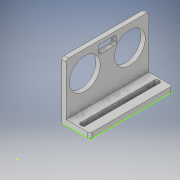
# Autodesk Inventor part: UltrasonicSensorMountSingle
Saved by Autodesk Inventor 2019 (Build 230136000, 136)
## iProperties
Created: 2020-06-23
Part Number: UltrasonicSensorMountSingle
Material: Generic
Document SubType Name: Modeling
Designer: garretthagen21
Density: 1 g/cm^3
Appearance: Default
Author: garretthagen21
Autodesk Inventor part; units mm, degrees
ref_plane "YZ Plane" through (0, 0, 0) normal (1, 0, 0) x (0, 1, 0)
ref_plane "XZ Plane" through (0, 0, 0) normal (0, 1, 0) x (-1, 0, 0)
ref_plane "XY Plane" through (0, 0, 0) normal (0, 0, 1) x (1, 0, 0)
sketch "Base" plane through (0, 0, 0) normal (0, 1, 0) x (-1, 0, 0)
  line L0 (-10.6945, -30.7069) -> (-10.6945, -77.3796)
  line L1 (5.3055, -77.3796) -> (5.3055, -30.7069)
  line L2 (5.3055, -30.7069) -> (-10.6945, -30.7069)
  line L3 (5.3055, -77.3796) -> (-10.6945, -77.3796)
  point P0 (0, 0)
  constraints: 8 end point, 1 horizontal, 1 parallel, 1 perpendicular
extrude "Extrusion1" add sketch "Base" along normal blind 3
sketch "FrontWall" plane through (0, 3, 0) normal (0, 1, 0) x (1, 0, 0)
  line L0 (-5.3055, 77.3796) -> (-5.3055, 30.7069) projected
  line L1 (-2.7655, 31.0004) -> (-2.7655, 77.0861)
  line L2 (-5.3055, 77.3796) -> (-2.7655, 77.3796)
  line L3 (10.6945, 77.3796) -> (-5.3055, 77.3796) projected
  line L4 (-2.7655, 77.0861) -> (-2.7655, 77.2936)
  line L5 (-2.7655, 77.2936) -> (-2.7655, 77.3796)
  line L6 (-2.7655, 31.0004) -> (-2.7655, 30.7069)
  line L7 (-5.3055, 30.7069) -> (-2.7655, 30.7069)
  line L8 (-5.3055, 30.7069) -> (10.6945, 30.7069) projected
  point P0 (0, 0)
  constraints: 12 end point, 2 collinear, 2 point on line, 1 vertical
extrude "Extrusion2" add sketch "FrontWall" along normal blind 29.464
sketch "Sketch5" plane through (-5.3055, 0, -77.3796) normal (-1, 0, 0) x (0, 0, 1)
  line L0 (-47.9308, 0) -> (-47.9308, 32.464)
  line L1 (0, 0) -> (0, 32.464)
  line L2 (46.1641, 31.6804) -> (0.7141, 31.6804)
  line L3 (0.7141, 31.6804) -> (0.7141, 10.0772)
  line L4 (0.7141, 10.0772) -> (46.1641, 10.0772)
  line L5 (46.1641, 10.0772) -> (46.1641, 31.6804)
  line L6 (23.4391, 30.4798) -> (18.3891, 30.4798)
  line L7 (18.3891, 30.4798) -> (18.3891, 25.6172)
  line L8 (18.3891, 25.6172) -> (28.4983, 25.6172)
  line L9 (28.4983, 25.6172) -> (28.4983, 30.4798)
  line L10 (28.4983, 30.4798) -> (23.4391, 30.4798)
  point P0 (77.3796, 0)
  point P1 (74.13, 0)
  point P2 (10.7141, 20.3272)
  point P3 (36.1565, 20.3272)
  dimension "d27" = 47.9308
  dimension "d28" = 45.45
  constraints: 22 end point, 5 perpendicular, 3 parallel, 1 horizontal, 1 point on line
  measures "d27" distance between parallel lines of L0 L1
  measures "d28" distance of L4.end L3.end
hole "Hole2" at (-5.3055, 20.3272, -41.2231) at (-5.3055, 20.3272, -66.6655) direction (1, 0, 0) diameter 17.5 end through all
extrude "Extrusion4" cut sketch "Sketch5" against normal blind 29.464 contours L10 L9 L8 L7 L6
fillet "Fillet1" radius 1.27 4 edges at (-4.0355, 30.4798, -58.9905) (-4.0355, 25.6172, -58.9905) (-4.0355, 30.4798, -48.8813) (-4.0355, 25.6172, -48.8813)
fillet "Fillet2" radius 1.27 4 edges at (-4.0355, 32.464, -30.7069) (-4.0355, 32.464, -77.3796) (10.6945, 1.5, -30.7069) (10.6945, 1.5, -77.3796)
sketch "Sketch8" plane through (0, 3, 0) normal (0, 1, 0) x (1, 0, 0)
  line L0 (3.818, 31.9431) -> (4.786, 31.9431)
  line L1 (5.802, 32.9591) -> (5.802, 75.143)
  line L2 (4.786, 76.159) -> (3.818, 76.159)
  line L3 (2.802, 75.143) -> (2.802, 32.9591)
  arc A0 (3.818, 76.159) -> (2.802, 75.143) centre (3.818, 75.143) ccw
  arc A1 (5.802, 75.143) -> (4.786, 76.159) centre (4.786, 75.143) ccw
  arc A2 (2.802, 32.9591) -> (3.818, 31.9431) centre (3.818, 32.9591) ccw
  arc A3 (4.786, 31.9431) -> (5.802, 32.9591) centre (4.786, 32.9591) ccw
  point P0 (0, 0)
  point P1 (5.802, 76.159)
  point P2 (2.802, 76.159)
  dimension "d62" = 3
  dimension "d63" = 1.016
  constraints: 8 end point, 8 point on circle, 8 tangent, 4 centre point, 4 point on line, 3 equal radius, 2 parallel, 1 horizontal, 1 perpendicular
  measures "d62" distance of point (2.802, 76.159) point (5.802, 76.159)
  measures "d63" radius of A0
extrude "Extrusion6" cut sketch "Sketch8" against normal through all
body "Solid1"
